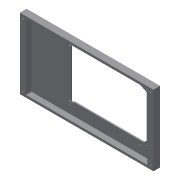
# Autodesk Inventor part: 04_OPENTRONS_Microscope_wellplate_base
Saved by Autodesk Inventor 2019.4 (Build 234330000, 330)
## iProperties
Created: 2020-11-05
Part Number: 04_OPENTRONS_Microscope_wellplate_base
Material: Generic
Document SubType Name: Modeling
Designer: diederichbenedict
Density: 1 g/cm^3
Appearance: Default
Author: diederichbenedict
Autodesk Inventor part; units mm, degrees
ref_plane "YZ Plane" through (0, 0, 0) normal (1, 0, 0) x (0, 1, 0)
ref_plane "XZ Plane" through (0, 0, 0) normal (0, 1, 0) x (-1, 0, 0)
ref_plane "XY Plane" through (0, 0, 0) normal (0, 0, 1) x (1, 0, 0)
sketch "Sketch1" plane through (0, 0, 0) normal (0, 0, 1) x (1, 0, 0)
  line L0 (55.6201, 39.7) -> (66.8, 34.5201)
  line L1 (66.8, 34.5201) -> (66.8, -34.5201)
  line L2 (66.8, -34.5201) -> (61.6201, -39.7)
  line L3 (61.6201, -39.7) -> (-54.2, -39.7)
  arc A0 (-58.8, -39.1) -> (-54.2, -39.7) centre (-56.5, -39.4) ccw
  line L4 (-58.8, -39.1) -> (-58.8, 39.1)
  arc A1 (-60.2, 39.7) -> (-58.8, 39.1) centre (-59.5, 39.4) ccw
  line L5 (-60.2, 39.7) -> (55.6201, 39.7)
  line L6 (-133.7, 52.7) -> (86.8, 52.7)
  line L7 (86.8, 52.7) -> (86.8, -63.9)
  line L8 (86.8, -63.9) -> (-133.7, -63.9)
  line L9 (-133.7, -63.9) -> (-133.7, 52.7)
  line L10 (-149.2, -74.9) -> (-149.2, -103.9) construction
  line L11 (86.8, -114.9) -> (86.8, -63.9) construction
  line L12 (-133.7, 52.7) -> (-133.7, -51.9) projected
  line L13 (-133.7, -63.9) -> (-123.7, -63.9) projected
  point P0 (0, 0)
  dimension "d5" = 13
  dimension "d15" = 0
  dimension "d47" = 0
  dimension "d50" = 0
  constraints: 20 end point, 4 point on circle, 2 centre point, 2 parallel, 1 horizontal, 1 perpendicular
  measures "d5" distance between parallel lines of L6 L5
  measures "d15" distance between parallel lines of L7 L11
  measures "d47" distance between parallel lines of L12 L9
  measures "d50" distance between parallel lines of L8 L13
extrude "Extrusion1" add sketch "Sketch1" along normal blind 2
hole "Hole1" at (66.7, 38.7385, 0) at (66.7, -40.9385, 0) at (55.2382, -45.8, 0) at (61.2382, 43.6, 0) at (-60.9, 38, 0) at (-60.9, -40.2, 0) at (-61.3, -45.8, 0) at (-55.3, 43.6, 0) direction (0, 0, 1) diameter 2.9 end through all
ref_plane "Work Plane3" through (-133.7, 41.6084, 11.0916) normal (0, 0, -1) x (0, 1, 0)
sketch "Sketch3" plane through (0, 0, 2) normal (0, 0, 1) x (1, 0, 0)
  circle A0 centre (-61.3, -45.8) radius 1.45 projected
  arc A1 (-60.2548, 39.2985) -> (-59.6015, 38.6452) centre (-60.9, 38) ccw projected
  circle A2 centre (55.2382, -45.8) radius 1.45 projected
  circle A3 centre (66.7, 38.7385) radius 1.45 projected
  circle A4 centre (66.7, -40.9385) radius 1.45 projected
  circle A5 centre (61.2382, 43.6) radius 1.45 projected
  circle A6 centre (-60.9, -40.2) radius 1.45 projected
  circle A7 centre (-55.3, 43.6) radius 1.45 projected
  line L0 (55.6201, 39.7) -> (66.8, 34.5201) projected
  line L1 (66.8, 34.5201) -> (66.8, -34.5201) projected
  line L2 (66.8, -34.5201) -> (61.6201, -39.7) projected
  line L3 (61.6201, -39.7) -> (-54.2, -39.7) projected
  arc A8 (-58.8, -39.1) -> (-54.2, -39.7) centre (-56.5, -39.4) ccw projected
  line L4 (-58.8, -39.1) -> (-58.8, 39.1) projected
  arc A9 (-59.6015, 38.6452) -> (-58.8, 39.1) centre (-59.5, 39.4) ccw projected
  line L5 (-60.2, 39.7) -> (55.6201, 39.7) projected
  line L6 (86.8, 52.7) -> (-133.7, 52.7) projected
  line L7 (-133.7, 52.7) -> (-133.7, -63.9) projected
  line L8 (-133.7, -63.9) -> (86.8, -63.9) projected
  line L9 (86.8, -63.9) -> (86.8, 52.7) projected
  line L10 (86.8, -63.9) -> (86.8, 52.7) projected
  line L11 (-133.7, 52.7) -> (-133.7, -63.9) projected
  line L12 (86.8, -63.9) -> (-133.7, -63.9)
  line L13 (-133.7, -63.9) -> (-133.7, -59.9)
  line L14 (-133.7, -59.9) -> (86.8, -59.9)
  line L15 (86.8, -59.9) -> (86.8, -63.9)
  line L16 (-133.7, 52.7) -> (86.8, 52.7)
  line L17 (86.8, 52.7) -> (86.8, 48.7)
  line L18 (86.8, 48.7) -> (-133.7, 48.7)
  line L19 (-133.7, 48.7) -> (-133.7, 52.7)
  arc A10 (-60.2, 39.7) -> (-60.2548, 39.2985) centre (-59.5, 39.4) ccw projected
  point P0 (0, 0)
  dimension "d17" = 4
  dimension "d18" = 4
  constraints: 16 end point, 4 parallel, 2 horizontal, 2 perpendicular, 2 point on line
  measures "d17" distance of L12.end L13.end
  measures "d18" distance of L16.end L17.end
extrude "Extrusion2" add sketch "Sketch3" along normal up to surface (9.0916 mm away) contours L9 L18 L7 L6 | L9 L8 L7 L14
sketch "Sketch8" plane through (0, 0, 2) normal (0, 0, 1) x (1, 0, 0)
  line L0 (-123.7, 52.7) -> (-123.7, -51.9) projected
  circle A0 centre (-128.7, 47.1542) radius 1.45 projected
  line L1 (76.8, 52.7) -> (76.8, -51.9) projected
  line L2 (86.8, -114.9) -> (86.8, 52.7) projected
  line L3 (-133.7, 52.7) -> (-133.7, -51.9) projected
  line L4 (-133.7, 52.7) -> (-123.7, 52.7)
  line L5 (-123.7, 52.7) -> (-123.7, -63.9)
  line L6 (-123.7, -63.9) -> (-133.7, -63.9)
  line L7 (-133.7, -63.9) -> (-133.7, 52.7)
  line L8 (86.8, -63.9) -> (-133.7, -63.9) projected
  line L9 (86.8, 52.7) -> (76.8, 52.7)
  line L10 (76.8, 52.7) -> (76.8, -63.9)
  line L11 (76.8, -63.9) -> (86.8, -63.9)
  line L12 (86.8, -63.9) -> (86.8, 52.7)
  point P0 (0, 0)
  constraints: 16 end point, 4 parallel, 4 point on line, 2 horizontal, 2 perpendicular
ref_plane "Work Plane2" through (-133.7, 41.6084, 11.0916) normal (0, 0, -1) x (0, 1, 0)
extrude "Extrusion5" add sketch "Sketch8" along normal up to surface (9.0916 mm away)
sketch "Sketch9" plane through (0, 0, 0) normal (0, 0, -1) x (-1, 0, 0)
  circle A0 centre (128.7, -57.3542) radius 1.45 projected
  circle A1 centre (128.7, 47.1542) radius 1.45 projected
  circle A2 centre (-81.8, -57.3542) radius 1.45 projected
  circle A3 centre (-81.8, 47.1542) radius 1.45 projected
  point P0 (0, 0)
extrude "Extrusion6" cut sketch "Sketch9" against normal through all
body "Solid1"
